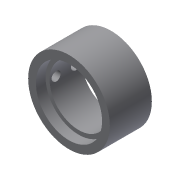
# Autodesk Inventor part: 30_focus_inlet_objective_mount_v7
Saved by Autodesk Inventor 2019.4 (Build 234330000, 330)
## iProperties
Created: 2019-10-25
Part Number: 30_focus_inlet_objective_mount_v7
Material: Generic
Document SubType Name: Modeling
Designer: marsikovabarbora
Density: 1 g/cm^3
Appearance: Default
Author: marsikovabarbora
Autodesk Inventor part; units mm, degrees
ref_plane "YZ Plane" through (0, 0, 0) normal (1, 0, 0) x (0, 1, 0)
ref_plane "XZ Plane" through (0, 0, 0) normal (0, 1, 0) x (-1, 0, 0)
ref_plane "XY Plane" through (0, 0, 0) normal (0, 0, 1) x (1, 0, 0)
sketch "Sketch1" plane through (0, 0, 0) normal (0, 0, 1) x (1, 0, 0)
  line L0 (9.6801, -14.008) -> (7.2052, -11.5331) construction
  line L1 (7.2052, -11.5331) -> (11.5893, -7.1491) construction
  line L2 (11.5893, -7.1491) -> (14.0642, -9.6239) construction
  line L3 (14.0642, -9.6239) -> (9.6801, -14.008) construction
  arc A0 (12.6369, -4.7496) -> (4.7496, -12.6369) centre (0, 0) ccw construction
  line L4 (10.9298, -3.0424) -> (12.6369, -4.7496) construction
  line L5 (11.6618, -4.6122) -> (10.9298, -3.0424) construction
  arc A1 (11.6618, -4.6122) -> (10.8551, -4.47) centre (11.2086, -4.8235) ccw construction
  line L6 (10.7915, -4.5335) -> (10.8551, -4.47) construction
  arc A2 (10.7915, -4.5335) -> (10.6527, -4.9738) centre (11.1451, -4.887) ccw construction
  line L7 (10.915, -6.4612) -> (10.6527, -4.9738) construction
  arc A3 (10.7761, -6.9016) -> (10.915, -6.4612) centre (10.4226, -6.548) ccw construction
  line L8 (6.9016, -10.7761) -> (10.7761, -6.9016) construction
  arc A4 (6.4612, -10.915) -> (6.9016, -10.7761) centre (6.548, -10.4226) ccw construction
  line L9 (6.4612, -10.915) -> (4.9738, -10.6527) construction
  arc A5 (4.9738, -10.6527) -> (4.5335, -10.7915) centre (4.887, -11.1451) ccw construction
  line L10 (4.5335, -10.7915) -> (4.47, -10.8551) construction
  arc A6 (4.47, -10.8551) -> (4.6122, -11.6618) centre (4.8235, -11.2086) ccw construction
  line L11 (4.6122, -11.6618) -> (3.0424, -10.9298) construction
  line L12 (3.0424, -10.9298) -> (4.7496, -12.6369) construction
  line L13 (-1.7167, -14.6498) -> (-1.7167, -17.5) construction
  line L14 (-1.7167, -17.5) -> (1.7167, -17.5) construction
  line L15 (1.7167, -14.6498) -> (1.7167, -17.5) construction
  arc A7 (1.7167, -14.6498) -> (6.9595, -13.0049) centre (0, 0) ccw construction
  arc A8 (6.9595, -13.0049) -> (8.2728, -15.1789) centre (8.2994, -13.6792) ccw construction
  line L16 (8.2728, -15.1789) -> (7.6816, -15.1684) construction
  arc A9 (8.5249, -17.8901) -> (7.6816, -15.1684) centre (7.655, -16.6682) ccw construction
  line L17 (8.5249, -17.8901) -> (13.5161, -14.3366) construction
  line L18 (13.5161, -14.3366) -> (13.5161, -12.2823) construction
  line L19 (13.5161, -12.2823) -> (14.6168, -12.2823) construction
  line L20 (14.6168, -12.2823) -> (14.6168, -1.9776) construction
  arc A10 (14.6168, -1.9776) -> (1.7167, 14.6498) centre (0, 0) ccw construction
  line L21 (1.7167, 14.6498) -> (1.7167, 17.5) construction
  line L22 (-1.7167, 17.5) -> (1.7167, 17.5) construction
  line L23 (-1.7167, 14.6498) -> (-1.7167, 17.5) construction
  arc A11 (-1.7167, 14.6498) -> (-14.2817, -3.6872) centre (0, 0) ccw construction
  line L24 (-14.2817, -3.6872) -> (-15.4135, -5.7935) construction
  arc A12 (-15.4135, -5.7935) -> (-14.5984, -8.502) centre (-13.6517, -6.7402) ccw construction
  line L25 (-14.5984, -8.502) -> (-9.6326, -11.1703) construction
  arc A13 (-9.6326, -11.1703) -> (-1.7167, -14.6498) centre (0, 0) ccw construction
  line L26 (-24.6, 24.6) -> (25.2, -25.2) construction
  line L27 (25.2, 24.6) -> (-24.6, -25.2) construction
  arc A14 (-1.4283, 10.15) -> (-9.5043, -3.8381) centre (0, 0) ccw
  circle A15 centre (0, 0) radius 10.1 construction
  line L28 (-1.4283, 10.15) -> (1.4283, 10.15)
  line L29 (-8.076, -6.3119) -> (-9.5043, -3.8381)
  line L30 (9.5043, -3.8381) -> (8.076, -6.3119)
  arc A16 (1.4283, 10.15) -> (-1.4283, 10.15) centre (0, 0) ccw
  arc A17 (9.5043, -3.8381) -> (1.4283, 10.15) centre (0, 0) ccw
  arc A18 (8.076, -6.3119) -> (9.5043, -3.8381) centre (0, 0) ccw
  arc A19 (-8.076, -6.3119) -> (8.076, -6.3119) centre (0, 0) ccw
  arc A20 (-9.5043, -3.8381) -> (-8.076, -6.3119) centre (0, 0) ccw
  arc A21 (10.7786, -4.5205) -> (10.6704, -4.6789) centre (11.1451, -4.887) ccw construction
  line L31 (10.7786, -4.5205) -> (10.8421, -4.457) construction
  arc A22 (11.7261, -4.7937) -> (10.8421, -4.457) centre (11.2086, -4.8235) ccw construction
  line L32 (11.7261, -4.7937) -> (10.8691, -2.9558) construction
  line L33 (10.8691, -2.9558) -> (12.6297, -4.7164) construction
  line L34 (4.7164, -12.6297) -> (2.9558, -10.8691) construction
  line L35 (2.9558, -10.8691) -> (4.4463, -11.5641) construction
  arc A23 (4.457, -10.8421) -> (4.4463, -11.5641) centre (4.8235, -11.2086) ccw construction
  line L36 (4.457, -10.8421) -> (4.5223, -10.7767) construction
  arc A24 (4.977, -10.6346) -> (4.6789, -10.6704) centre (4.887, -11.1451) ccw
  arc A25 (4.6789, -10.6704) -> (4.5223, -10.7767) centre (4.887, -11.1451) ccw construction
  arc A26 (10.6704, -4.6789) -> (10.6346, -4.977) centre (11.1451, -4.887) ccw
  circle A27 centre (0, 0) radius 12.65
  dimension "d4" = 20.2
  dimension "d5" = 10.15
  dimension "d6" = 20.5
  dimension "d9" = 360
  dimension "d28" = 25.3
  constraints: 24 point on circle, 18 end point, 14 centre point, 3 coincident, 1 horizontal, 16 other
  measures "d4" diameter of A15
  measures "d5" distance from line of L28 point (0, 0)
  measures "d6" diameter of A14
  measures "d28" diameter of A27
extrude "Extrusion1" add sketch "Sketch1" against normal blind 3
sketch "Sketch3" plane through (0, 0, -3) normal (0, 0, -1) x (-1, 0, 0)
  circle A0 centre (0, 0) radius 10.25 projected
  circle A1 centre (0, 0) radius 9
  circle A2 centre (0, 0) radius 11.5312
  circle A3 centre (0, 0) radius 12.65 projected
  dimension "d17" = 18
  constraints: 2 centre point, 1 coincident
  measures "d17" diameter of A1
extrude "Extrusion3" add sketch "Sketch3" along normal blind 10 contours A0 | A2 | A3
sketch "Sketch4" plane through (0, -10.7054, 0) normal (1, 0, 0) x (0, 0, -1)
  line L0 (13, 19.7054) -> (13, 1.7054) projected
  line L1 (3, 1.7054) -> (3, 19.7054) projected
  circle A0 centre (11, 10.7054) radius 1.4
  circle A1 centre (5, 10.7054) radius 1.4
  dimension "d24" = 2.8
  dimension "d25" = 2.8
  dimension "d26" = 6
  dimension "d27" = 2
  constraints: 2 centre point
  measures "d24" diameter of A0
  measures "d25" diameter of A1
  measures "d26" distance of A0.centre A1.centre
  measures "d27" distance from line of A1.centre L1
extrude "Extrusion4" cut sketch "Sketch4" against normal through all
body "Solid1"
